Autodesk Fusion 360 part; units mm, degrees
(part 2 of 3)
sketch "Knuckle (2) (2)" plane through (0, 0, 0) normal (1, 0, 0) x (0, 0, -1) in component "Wedgelet_Block_PETG_R"
  line L0 (100, 11) -> (100, 16.5)
  line L1 (100, 16.5) -> (104, 16.5)
  line L2 (104, 16.5) -> (104, 11)
  line L3 (104, 11) -> (100, 11)
extrude "Extrude4'''''" add sketch "Knuckle (2) (2)" along normal blind 4 from surface at 84 bodies 28 in component "Wedgelet_Block_PETG_R"
sketch "Bridge (2)" plane through (0, 0, 0) normal (1, 0, 0) x (0, 0, -1) in component "Wedgelet_Block_PETG_R"
  line L0 (97, 7) -> (97, 10)
  line L1 (97, 10) -> (101, 10)
  line L2 (101, 10) -> (101, 7)
  line L3 (101, 7) -> (97, 7)
extrude "Extrude5'''''" add sketch "Bridge (2)" along normal blind 10 from surface at 70 bodies 28 in component "Wedgelet_Block_PETG_R"
sketch "Rail (2)" plane through (0, 0, 0) normal (1, 0, 0) x (0, 0, -1) in component "Wedgelet_Block_PETG_R"
  line L0 (64, 7) -> (64, 18)
  line L1 (64, 18) -> (98, 18)
  line L2 (98, 18) -> (98, 7)
  line L3 (98, 7) -> (64, 7)
extrude "Extrude6'''''" add sketch "Rail (2)" along normal blind 10 from surface at 70 bodies 28 in component "Wedgelet_Block_PETG_R"
sketch "Pin_Bore (4)" plane through (0, 0, 0) normal (1, 0, 0) x (0, 0, -1) in component "Wedgelet_Block_PETG_R"
  circle A0 centre (102, 14.5) radius 1.6
extrude "Extrude7''''" cut sketch "Pin_Bore (4)" along normal blind 56 from surface at 33 bodies 28 in component "Wedgelet_Block_PETG_R"
sketch "Wall_Insert (2)" plane through (0, 0, 0) normal (1, 0, 0) x (0, 0, -1) in component "Wedgelet_Block_PETG_R"
  circle A0 centre (80, 13.5) radius 2
extrude "Extrude8''''" cut sketch "Wall_Insert (2)" along normal blind 8 from surface at 72 bodies 28 in component "Wedgelet_Block_PETG_R"
sketch "Wall_Insert (1) (2)" plane through (0, 0, 0) normal (1, 0, 0) x (0, 0, -1) in component "Wedgelet_Block_PETG_R"
  circle A0 centre (92, 13.5) radius 2
extrude "Extrude9''''" cut sketch "Wall_Insert (1) (2)" along normal blind 8 from surface at 72 bodies 28 in component "Wedgelet_Block_PETG_R"
sketch "Wedgelet_Carrier_PETG_R1" plane through (0, 0, 0) normal (1, 0, 0) x (0, 0, -1) in component "Wedgelet_Carrier_PETG_R1"
  line L0 (100, 11.5) -> (100, 20.5)
  line L1 (100, 20.5) -> (114, 10.5)
  line L2 (114, 10.5) -> (114, 8)
  line L3 (114, 8) -> (105, 8)
  line L4 (105, 8) -> (104.5, 11.5)
  line L5 (104.5, 11.5) -> (100, 11.5)
extrude "Extrude1''''''''''''''''''''''''''''" add sketch "Wedgelet_Carrier_PETG_R1" along normal blind 20 from surface at 39 separate body makes body 29 in component "Wedgelet_Carrier_PETG_R1"
sketch "Pin_Bore (5)" plane through (0, 0, 0) normal (1, 0, 0) x (0, 0, -1) in component "Wedgelet_Carrier_PETG_R1"
  circle A0 centre (102, 14.5) radius 1.6
extrude "Extrude2'''''''''''''" cut sketch "Pin_Bore (5)" along normal blind 22 from surface at 38 bodies 29 in component "Wedgelet_Carrier_PETG_R1"
sketch "Wedgelet_Insert (3)" plane through (0, 60.8716, -43.4797) normal (0, 0.813733, -0.581238) x (0, 0.581238, 0.813733) in component "Wedgelet_Carrier_PETG_R1"
  line L0 (-86.6626, 39) -> (-69.458, 39)
  line L1 (-69.458, 39) -> (-69.458, 59)
  line L2 (-69.458, 59) -> (-86.6626, 59)
  line L3 (-86.6626, 59) -> (-86.6626, 39)
  circle A0 through (-78.5829, 49, -0.0046) (-81.5829, 50.7321, -0.0046) (-81.5829, 47.2679, -0.0046)
extrude "Extrude3''''''''''" cut sketch "Wedgelet_Insert (3)" along normal mid plane 12 contours A0 in plane through (0, 60.8679, -43.4771) normal (0, 0.813733, -0.581238) bodies 29 in component "Wedgelet_Carrier_PETG_R1"
sketch "Wedgelet_Carrier_PETG_R2" plane through (0, 0, 0) normal (1, 0, 0) x (0, 0, -1) in component "Wedgelet_Carrier_PETG_R2"
  line L0 (100, 11.5) -> (100, 20.5)
  line L1 (100, 20.5) -> (114, 10.5)
  line L2 (114, 10.5) -> (114, 8)
  line L3 (114, 8) -> (105, 8)
  line L4 (105, 8) -> (104.5, 11.5)
  line L5 (104.5, 11.5) -> (100, 11.5)
extrude "Extrude1'''''''''''''''''''''''''''''" add sketch "Wedgelet_Carrier_PETG_R2" along normal blind 16 from surface at 67 separate body makes body 30 in component "Wedgelet_Carrier_PETG_R2"
sketch "Pin_Bore (6)" plane through (0, 0, 0) normal (1, 0, 0) x (0, 0, -1) in component "Wedgelet_Carrier_PETG_R2"
  circle A0 centre (102, 14.5) radius 1.6
extrude "Extrude2''''''''''''''" cut sketch "Pin_Bore (6)" along normal blind 18 from surface at 66 bodies 30 in component "Wedgelet_Carrier_PETG_R2"
sketch "Wedgelet_Insert (4)" plane through (0, 60.8716, -43.4797) normal (0, 0.813733, -0.581238) x (0, 0.581238, 0.813733) in component "Wedgelet_Carrier_PETG_R2"
  line L0 (-86.6626, 67) -> (-69.458, 67)
  line L1 (-69.458, 67) -> (-69.458, 83)
  line L2 (-69.458, 83) -> (-86.6626, 83)
  line L3 (-86.6626, 83) -> (-86.6626, 67)
  circle A0 through (-78.5829, 75, -0.0046) (-81.5829, 76.7321, -0.0046) (-81.5829, 73.2679, -0.0046)
extrude "Extrude3'''''''''''" cut sketch "Wedgelet_Insert (4)" along normal mid plane 12 contours A0 in plane through (0, 60.8679, -43.4771) normal (0, 0.813733, -0.581238) bodies 30 in component "Wedgelet_Carrier_PETG_R2"
sketch "Hinge_Pin_D3_R" plane through (0, 0, 0) normal (1, 0, 0) x (0, 0, -1) in component "Hinge_Pin_D3_R"
  circle A0 centre (102, 14.5) radius 1.5
extrude "Extrude1''''''''''''''''''''''''''''''" add sketch "Hinge_Pin_D3_R" along normal blind 57 from surface at 33.5 separate body makes body 31 in component "Hinge_Pin_D3_R"
sketch "Eclip_Groove (2)" plane through (0, 0, 0) normal (1, 0, 0) x (0, 0, -1) in component "Hinge_Pin_D3_R"
  circle A0 centre (102, 14.5) radius 1.5
  circle A1 centre (102, 14.5) radius 1.15
extrude "Extrude2'''''''''''''''" cut sketch "Eclip_Groove (2)" along normal blind 0.6 from surface at 89 bodies 31 in component "Hinge_Pin_D3_R"
sketch "Eclip_DIN6799_2.3_R" plane through (0, 0, 0) normal (1, 0, 0) x (0, 0, -1) in component "Eclip_DIN6799_2.3_R"
  circle A0 centre (102, 14.5) radius 3.5
  circle A1 centre (102, 14.5) radius 1.15
extrude "Extrude1'''''''''''''''''''''''''''''''" add sketch "Eclip_DIN6799_2.3_R" along normal blind 0.6 from surface at 89 separate body makes body 32 in component "Eclip_DIN6799_2.3_R"
sketch "Sketch1 (8)" plane through (0, 0, 0) normal (0, 1, 0) x (1, 0, 0) in component "Skirt_Plate_1mm_L"
  line L0 (-89.5, -110) -> (-88.5, -110)
  line L1 (-88.5, -110) -> (-88.5, 97)
  line L2 (-88.5, 97) -> (-89.5, 97)
  line L3 (-89.5, 97) -> (-89.5, -110)
extrude "Extrude1''''''''''''''''''''''''''''''''" add sketch "Sketch1 (8)" along normal blind 13 separate body makes body 33 in component "Skirt_Plate_1mm_L"
sketch "Skirt_Wire_D1.5_L" plane through (0, 0, 0) normal (0, 0, 1) x (1, 0, 0) in component "Skirt_Wire_D1.5_L"
  circle A0 centre (-90, 15) radius 0.75
extrude "Extrude1'''''''''''''''''''''''''''''''''" add sketch "Skirt_Wire_D1.5_L" along normal blind 207 from surface at -97 separate body makes body 34 in component "Skirt_Wire_D1.5_L"
sketch "Skirt_Knuckle" plane through (0, 0, 0) normal (1, 0, 0) x (0, 0, -1) in component "Tub_TPU"
  line L0 (-108, 13) -> (-108, 17)
  line L1 (-108, 17) -> (-98, 17)
  line L2 (-98, 17) -> (-98, 13)
  line L3 (-98, 13) -> (-108, 13)
extrude "Extrude42" add sketch "Skirt_Knuckle" along normal blind 4 from surface at -92 bodies 1 in component "Tub_TPU"
sketch "Skirt_Knuckle (1)" plane through (0, 0, 0) normal (1, 0, 0) x (0, 0, -1) in component "Tub_TPU"
  line L0 (-55, 13) -> (-55, 17)
  line L1 (-55, 17) -> (-45, 17)
  line L2 (-45, 17) -> (-45, 13)
  line L3 (-45, 13) -> (-55, 13)
extrude "Extrude43" add sketch "Skirt_Knuckle (1)" along normal blind 4 from surface at -92 bodies 1 in component "Tub_TPU"
sketch "Skirt_Knuckle (2)" plane through (0, 0, 0) normal (1, 0, 0) x (0, 0, -1) in component "Tub_TPU"
  line L0 (0, 13) -> (0, 17)
  line L1 (0, 17) -> (10, 17)
  line L2 (10, 17) -> (10, 13)
  line L3 (10, 13) -> (0, 13)
extrude "Extrude44" add sketch "Skirt_Knuckle (2)" along normal blind 4 from surface at -92 bodies 1 in component "Tub_TPU"
sketch "Skirt_Knuckle (3)" plane through (0, 0, 0) normal (1, 0, 0) x (0, 0, -1) in component "Tub_TPU"
  line L0 (80, 13) -> (80, 17)
  line L1 (80, 17) -> (90, 17)
  line L2 (90, 17) -> (90, 13)
  line L3 (90, 13) -> (80, 13)
extrude "Extrude45" add sketch "Skirt_Knuckle (3)" along normal blind 4 from surface at -92 bodies 1 in component "Tub_TPU"
sketch "Skirt_Wire_Bore" plane through (0, 0, 0) normal (0, 0, 1) x (1, 0, 0) in component "Tub_TPU"
  circle A0 centre (-90, 15) radius 0.8
extrude "Extrude46" cut sketch "Skirt_Wire_Bore" along normal blind 209 from surface at -98 bodies 1 in component "Tub_TPU"
sketch "Sketch1 (9)" plane through (0, 0, 0) normal (0, 1, 0) x (1, 0, 0) in component "Skirt_Clip_PETG_L1"
  line L0 (-92, -90) -> (-89.5, -90)
  line L1 (-89.5, -90) -> (-89.5, -75)
  line L2 (-89.5, -75) -> (-92, -75)
  line L3 (-92, -75) -> (-92, -90)
extrude "Extrude1''''''''''''''''''''''''''''''''''" add sketch "Sketch1 (9)" along normal blind 7 from surface at 10 separate body makes body 35 in component "Skirt_Clip_PETG_L1"
sketch "Wire_Bore" plane through (0, 0, 0) normal (0, 0, 1) x (1, 0, 0) in component "Skirt_Clip_PETG_L1"
  circle A0 centre (-90, 15) radius 0.8
extrude "Extrude2''''''''''''''''" cut sketch "Wire_Bore" along normal blind 17 from surface at 74 bodies 35 in component "Skirt_Clip_PETG_L1"
sketch "M2_Hole" plane through (0, 0, 0) normal (1, 0, 0) x (0, 0, -1) in component "Skirt_Clip_PETG_L1"
  circle A0 centre (-82.5, 11.5) radius 1.1
extrude "Extrude3''''''''''''" cut sketch "M2_Hole" along normal blind 5 from surface at -93 bodies 35 in component "Skirt_Clip_PETG_L1"
sketch "M2_Hole (2)" plane through (0, 0, 0) normal (1, 0, 0) x (0, 0, -1) in component "Skirt_Plate_1mm_L"
  circle A0 centre (-82.5, 11.5) radius 1.1
extrude "Extrude2'''''''''''''''''" cut sketch "M2_Hole (2)" along normal blind 5 from surface at -93 bodies 33 in component "Skirt_Plate_1mm_L"
sketch "Sketch1 (10)" plane through (0, 0, 0) normal (0, 1, 0) x (1, 0, 0) in component "Skirt_Clip_PETG_L2"
  line L0 (-92, -35) -> (-89.5, -35)
  line L1 (-89.5, -35) -> (-89.5, -20)
  line L2 (-89.5, -20) -> (-92, -20)
  line L3 (-92, -20) -> (-92, -35)
extrude "Extrude1'''''''''''''''''''''''''''''''''''" add sketch "Sketch1 (10)" along normal blind 7 from surface at 10 separate body makes body 36 in component "Skirt_Clip_PETG_L2"
sketch "Wire_Bore (2)" plane through (0, 0, 0) normal (0, 0, 1) x (1, 0, 0) in component "Skirt_Clip_PETG_L2"
  circle A0 centre (-90, 15) radius 0.8
extrude "Extrude2''''''''''''''''''" cut sketch "Wire_Bore (2)" along normal blind 17 from surface at 19 bodies 36 in component "Skirt_Clip_PETG_L2"
sketch "M2_Hole (3)" plane through (0, 0, 0) normal (1, 0, 0) x (0, 0, -1) in component "Skirt_Clip_PETG_L2"
  circle A0 centre (-27.5, 11.5) radius 1.1
extrude "Extrude3'''''''''''''" cut sketch "M2_Hole (3)" along normal blind 5 from surface at -93 bodies 36 in component "Skirt_Clip_PETG_L2"
sketch "M2_Hole (1)" plane through (0, 0, 0) normal (1, 0, 0) x (0, 0, -1) in component "Skirt_Plate_1mm_L"
  circle A0 centre (-27.5, 11.5) radius 1.1
extrude "Extrude3''''''''''''''" cut sketch "M2_Hole (1)" along normal blind 5 from surface at -93 bodies 33 in component "Skirt_Plate_1mm_L"
sketch "Sketch1 (11)" plane through (0, 0, 0) normal (0, 1, 0) x (1, 0, 0) in component "Skirt_Clip_PETG_L3"
  line L0 (-92, 25) -> (-89.5, 25)
  line L1 (-89.5, 25) -> (-89.5, 40)
  line L2 (-89.5, 40) -> (-92, 40)
  line L3 (-92, 40) -> (-92, 25)
extrude "Extrude1''''''''''''''''''''''''''''''''''''" add sketch "Sketch1 (11)" along normal blind 7 from surface at 10 separate body makes body 37 in component "Skirt_Clip_PETG_L3"
sketch "Wire_Bore (3)" plane through (0, 0, 0) normal (0, 0, 1) x (1, 0, 0) in component "Skirt_Clip_PETG_L3"
  circle A0 centre (-90, 15) radius 0.8
extrude "Extrude2'''''''''''''''''''" cut sketch "Wire_Bore (3)" along normal blind 17 from surface at -41 bodies 37 in component "Skirt_Clip_PETG_L3"
sketch "M2_Hole (4)" plane through (0, 0, 0) normal (1, 0, 0) x (0, 0, -1) in component "Skirt_Clip_PETG_L3"
  circle A0 centre (32.5, 11.5) radius 1.1
extrude "Extrude3'''''''''''''''" cut sketch "M2_Hole (4)" along normal blind 5 from surface at -93 bodies 37 in component "Skirt_Clip_PETG_L3"
sketch "M2_Hole (2) (2)" plane through (0, 0, 0) normal (1, 0, 0) x (0, 0, -1) in component "Skirt_Plate_1mm_L"
  circle A0 centre (32.5, 11.5) radius 1.1
extrude "Extrude4''''''" cut sketch "M2_Hole (2) (2)" along normal blind 5 from surface at -93 bodies 33 in component "Skirt_Plate_1mm_L"
sketch "Sketch1 (12)" plane through (0, 0, 0) normal (0, 1, 0) x (1, 0, 0) in component "Skirt_Clip_PETG_L4"
  line L0 (-92, 55) -> (-89.5, 55)
  line L1 (-89.5, 55) -> (-89.5, 70)
  line L2 (-89.5, 70) -> (-92, 70)
  line L3 (-92, 70) -> (-92, 55)
extrude "Extrude1'''''''''''''''''''''''''''''''''''''" add sketch "Sketch1 (12)" along normal blind 7 from surface at 10 separate body makes body 38 in component "Skirt_Clip_PETG_L4"
sketch "Wire_Bore (4)" plane through (0, 0, 0) normal (0, 0, 1) x (1, 0, 0) in component "Skirt_Clip_PETG_L4"
  circle A0 centre (-90, 15) radius 0.8
extrude "Extrude2''''''''''''''''''''" cut sketch "Wire_Bore (4)" along normal blind 17 from surface at -71 bodies 38 in component "Skirt_Clip_PETG_L4"
sketch "M2_Hole (5)" plane through (0, 0, 0) normal (1, 0, 0) x (0, 0, -1) in component "Skirt_Clip_PETG_L4"
  circle A0 centre (62.5, 11.5) radius 1.1
extrude "Extrude3''''''''''''''''" cut sketch "M2_Hole (5)" along normal blind 5 from surface at -93 bodies 38 in component "Skirt_Clip_PETG_L4"
sketch "M2_Hole (3) (2)" plane through (0, 0, 0) normal (1, 0, 0) x (0, 0, -1) in component "Skirt_Plate_1mm_L"
  circle A0 centre (62.5, 11.5) radius 1.1
extrude "Extrude5''''''" cut sketch "M2_Hole (3) (2)" along normal blind 5 from surface at -93 bodies 33 in component "Skirt_Plate_1mm_L"
sketch "Sketch1 (13)" plane through (0, 0, 0) normal (0, 1, 0) x (1, 0, 0) in component "Skirt_Plate_1mm_R"
  line L0 (88.5, -110) -> (89.5, -110)
  line L1 (89.5, -110) -> (89.5, 97)
  line L2 (89.5, 97) -> (88.5, 97)
  line L3 (88.5, 97) -> (88.5, -110)
extrude "Extrude1''''''''''''''''''''''''''''''''''''''" add sketch "Sketch1 (13)" along normal blind 13 separate body makes body 39 in component "Skirt_Plate_1mm_R"
sketch "Skirt_Wire_D1.5_R" plane through (0, 0, 0) normal (0, 0, 1) x (1, 0, 0) in component "Skirt_Wire_D1.5_R"
  circle A0 centre (90, 15) radius 0.75
extrude "Extrude1'''''''''''''''''''''''''''''''''''''''" add sketch "Skirt_Wire_D1.5_R" along normal blind 207 from surface at -97 separate body makes body 40 in component "Skirt_Wire_D1.5_R"
sketch "Skirt_Knuckle (4)" plane through (0, 0, 0) normal (1, 0, 0) x (0, 0, -1) in component "Tub_TPU"
  line L0 (-108, 13) -> (-108, 17)
  line L1 (-108, 17) -> (-98, 17)
  line L2 (-98, 17) -> (-98, 13)
  line L3 (-98, 13) -> (-108, 13)
extrude "Extrude47" add sketch "Skirt_Knuckle (4)" along normal blind 4 from surface at 88 bodies 1 in component "Tub_TPU"
sketch "Skirt_Knuckle (5)" plane through (0, 0, 0) normal (1, 0, 0) x (0, 0, -1) in component "Tub_TPU"
  line L0 (-55, 13) -> (-55, 17)
  line L1 (-55, 17) -> (-45, 17)
  line L2 (-45, 17) -> (-45, 13)
  line L3 (-45, 13) -> (-55, 13)
extrude "Extrude48" add sketch "Skirt_Knuckle (5)" along normal blind 4 from surface at 88 bodies 1 in component "Tub_TPU"
sketch "Skirt_Knuckle (6)" plane through (0, 0, 0) normal (1, 0, 0) x (0, 0, -1) in component "Tub_TPU"
  line L0 (0, 13) -> (0, 17)
  line L1 (0, 17) -> (10, 17)
  line L2 (10, 17) -> (10, 13)
  line L3 (10, 13) -> (0, 13)
extrude "Extrude49" add sketch "Skirt_Knuckle (6)" along normal blind 4 from surface at 88 bodies 1 in component "Tub_TPU"
sketch "Skirt_Knuckle (7)" plane through (0, 0, 0) normal (1, 0, 0) x (0, 0, -1) in component "Tub_TPU"
  line L0 (80, 13) -> (80, 17)
  line L1 (80, 17) -> (90, 17)
  line L2 (90, 17) -> (90, 13)
  line L3 (90, 13) -> (80, 13)
extrude "Extrude50" add sketch "Skirt_Knuckle (7)" along normal blind 4 from surface at 88 bodies 1 in component "Tub_TPU"
sketch "Skirt_Wire_Bore (1)" plane through (0, 0, 0) normal (0, 0, 1) x (1, 0, 0) in component "Tub_TPU"
  circle A0 centre (90, 15) radius 0.8
extrude "Extrude51" cut sketch "Skirt_Wire_Bore (1)" along normal blind 209 from surface at -98 bodies 1 in component "Tub_TPU"
sketch "Sketch1 (14)" plane through (0, 0, 0) normal (0, 1, 0) x (1, 0, 0) in component "Skirt_Clip_PETG_R1"
  line L0 (89.5, -90) -> (92, -90)
  line L1 (92, -90) -> (92, -75)
  line L2 (92, -75) -> (89.5, -75)
  line L3 (89.5, -75) -> (89.5, -90)
extrude "Extrude1''''''''''''''''''''''''''''''''''''''''" add sketch "Sketch1 (14)" along normal blind 7 from surface at 10 separate body makes body 41 in component "Skirt_Clip_PETG_R1"
sketch "Wire_Bore (5)" plane through (0, 0, 0) normal (0, 0, 1) x (1, 0, 0) in component "Skirt_Clip_PETG_R1"
  circle A0 centre (90, 15) radius 0.8
extrude "Extrude2'''''''''''''''''''''" cut sketch "Wire_Bore (5)" along normal blind 17 from surface at 74 bodies 41 in component "Skirt_Clip_PETG_R1"
sketch "M2_Hole (6)" plane through (0, 0, 0) normal (1, 0, 0) x (0, 0, -1) in component "Skirt_Clip_PETG_R1"
  circle A0 centre (-82.5, 11.5) radius 1.1
extrude "Extrude3'''''''''''''''''" cut sketch "M2_Hole (6)" along normal blind 5 from surface at 88 bodies 41 in component "Skirt_Clip_PETG_R1"
sketch "M2_Hole (7)" plane through (0, 0, 0) normal (1, 0, 0) x (0, 0, -1) in component "Skirt_Plate_1mm_R"
  circle A0 centre (-82.5, 11.5) radius 1.1
extrude "Extrude2''''''''''''''''''''''" cut sketch "M2_Hole (7)" along normal blind 5 from surface at 88 bodies 39 in component "Skirt_Plate_1mm_R"
sketch "Sketch1 (15)" plane through (0, 0, 0) normal (0, 1, 0) x (1, 0, 0) in component "Skirt_Clip_PETG_R2"
  line L0 (89.5, -35) -> (92, -35)
  line L1 (92, -35) -> (92, -20)
  line L2 (92, -20) -> (89.5, -20)
  line L3 (89.5, -20) -> (89.5, -35)
extrude "Extrude1'''''''''''''''''''''''''''''''''''''''''" add sketch "Sketch1 (15)" along normal blind 7 from surface at 10 separate body makes body 42 in component "Skirt_Clip_PETG_R2"
sketch "Wire_Bore (6)" plane through (0, 0, 0) normal (0, 0, 1) x (1, 0, 0) in component "Skirt_Clip_PETG_R2"
  circle A0 centre (90, 15) radius 0.8
extrude "Extrude2'''''''''''''''''''''''" cut sketch "Wire_Bore (6)" along normal blind 17 from surface at 19 bodies 42 in component "Skirt_Clip_PETG_R2"
sketch "M2_Hole (8)" plane through (0, 0, 0) normal (1, 0, 0) x (0, 0, -1) in component "Skirt_Clip_PETG_R2"
  circle A0 centre (-27.5, 11.5) radius 1.1
extrude "Extrude3''''''''''''''''''" cut sketch "M2_Hole (8)" along normal blind 5 from surface at 88 bodies 42 in component "Skirt_Clip_PETG_R2"
sketch "M2_Hole (1) (2)" plane through (0, 0, 0) normal (1, 0, 0) x (0, 0, -1) in component "Skirt_Plate_1mm_R"
  circle A0 centre (-27.5, 11.5) radius 1.1
extrude "Extrude3'''''''''''''''''''" cut sketch "M2_Hole (1) (2)" along normal blind 5 from surface at 88 bodies 39 in component "Skirt_Plate_1mm_R"
sketch "Sketch1 (16)" plane through (0, 0, 0) normal (0, 1, 0) x (1, 0, 0) in component "Skirt_Clip_PETG_R3"
  line L0 (89.5, 25) -> (92, 25)
  line L1 (92, 25) -> (92, 40)
  line L2 (92, 40) -> (89.5, 40)
  line L3 (89.5, 40) -> (89.5, 25)
extrude "Extrude1''''''''''''''''''''''''''''''''''''''''''" add sketch "Sketch1 (16)" along normal blind 7 from surface at 10 separate body makes body 43 in component "Skirt_Clip_PETG_R3"
sketch "Wire_Bore (7)" plane through (0, 0, 0) normal (0, 0, 1) x (1, 0, 0) in component "Skirt_Clip_PETG_R3"
  circle A0 centre (90, 15) radius 0.8
extrude "Extrude2''''''''''''''''''''''''" cut sketch "Wire_Bore (7)" along normal blind 17 from surface at -41 bodies 43 in component "Skirt_Clip_PETG_R3"
sketch "M2_Hole (9)" plane through (0, 0, 0) normal (1, 0, 0) x (0, 0, -1) in component "Skirt_Clip_PETG_R3"
  circle A0 centre (32.5, 11.5) radius 1.1
extrude "Extrude3''''''''''''''''''''" cut sketch "M2_Hole (9)" along normal blind 5 from surface at 88 bodies 43 in component "Skirt_Clip_PETG_R3"
sketch "M2_Hole (2) (3)" plane through (0, 0, 0) normal (1, 0, 0) x (0, 0, -1) in component "Skirt_Plate_1mm_R"
  circle A0 centre (32.5, 11.5) radius 1.1
extrude "Extrude4'''''''" cut sketch "M2_Hole (2) (3)" along normal blind 5 from surface at 88 bodies 39 in component "Skirt_Plate_1mm_R"
sketch "Sketch1 (17)" plane through (0, 0, 0) normal (0, 1, 0) x (1, 0, 0) in component "Skirt_Clip_PETG_R4"
  line L0 (89.5, 55) -> (92, 55)
  line L1 (92, 55) -> (92, 70)
  line L2 (92, 70) -> (89.5, 70)
  line L3 (89.5, 70) -> (89.5, 55)
extrude "Extrude1'''''''''''''''''''''''''''''''''''''''''''" add sketch "Sketch1 (17)" along normal blind 7 from surface at 10 separate body makes body 44 in component "Skirt_Clip_PETG_R4"
sketch "Wire_Bore (8)" plane through (0, 0, 0) normal (0, 0, 1) x (1, 0, 0) in component "Skirt_Clip_PETG_R4"
  circle A0 centre (90, 15) radius 0.8
extrude "Extrude2'''''''''''''''''''''''''" cut sketch "Wire_Bore (8)" along normal blind 17 from surface at -71 bodies 44 in component "Skirt_Clip_PETG_R4"
sketch "M2_Hole (10)" plane through (0, 0, 0) normal (1, 0, 0) x (0, 0, -1) in component "Skirt_Clip_PETG_R4"
  circle A0 centre (62.5, 11.5) radius 1.1
extrude "Extrude3'''''''''''''''''''''" cut sketch "M2_Hole (10)" along normal blind 5 from surface at 88 bodies 44 in component "Skirt_Clip_PETG_R4"
sketch "M2_Hole (3) (3)" plane through (0, 0, 0) normal (1, 0, 0) x (0, 0, -1) in component "Skirt_Plate_1mm_R"
  circle A0 centre (62.5, 11.5) radius 1.1
extrude "Extrude5'''''''" cut sketch "M2_Hole (3) (3)" along normal blind 5 from surface at 88 bodies 39 in component "Skirt_Plate_1mm_R"
sketch "Sketch1 (18)" plane through (0, 0, 0) normal (0, 1, 0) x (1, 0, 0) in component "Skirt_Plate_1mm_Rear"
  line L0 (-88, -111.5) -> (88, -111.5)
  line L1 (88, -111.5) -> (88, -110.5)
  line L2 (88, -110.5) -> (-88, -110.5)
  line L3 (-88, -110.5) -> (-88, -111.5)
extrude "Extrude1''''''''''''''''''''''''''''''''''''''''''''" add sketch "Sketch1 (18)" along normal blind 13 separate body makes body 45 in component "Skirt_Plate_1mm_Rear"
sketch "Skirt_Wire_D1.5_Rear" plane through (0, 0, 0) normal (1, 0, 0) x (0, 0, -1) in component "Skirt_Wire_D1.5_Rear"
  circle A0 centre (-112, 15) radius 0.75
extrude "Extrude1'''''''''''''''''''''''''''''''''''''''''''''" add sketch "Skirt_Wire_D1.5_Rear" along normal blind 176 from surface at -88 separate body makes body 46 in component "Skirt_Wire_D1.5_Rear"
sketch "Skirt_Knuckle (8)" plane through (0, 0, 0) normal (1, 0, 0) x (0, 0, -1) in component "Tub_TPU"
  line L0 (-114, 13) -> (-114, 17)
  line L1 (-114, 17) -> (-110, 17)
  line L2 (-110, 17) -> (-110, 13)
  line L3 (-110, 13) -> (-114, 13)
extrude "Extrude52" add sketch "Skirt_Knuckle (8)" along normal blind 10 from surface at -86 bodies 1 in component "Tub_TPU"
sketch "Skirt_Knuckle (9)" plane through (0, 0, 0) normal (1, 0, 0) x (0, 0, -1) in component "Tub_TPU"
  line L0 (-114, 13) -> (-114, 17)
  line L1 (-114, 17) -> (-110, 17)
  line L2 (-110, 17) -> (-110, 13)
  line L3 (-110, 13) -> (-114, 13)
extrude "Extrude53" add sketch "Skirt_Knuckle (9)" along normal blind 10 from surface at -30 bodies 1 in component "Tub_TPU"
sketch "Skirt_Knuckle (10)" plane through (0, 0, 0) normal (1, 0, 0) x (0, 0, -1) in component "Tub_TPU"
  line L0 (-114, 13) -> (-114, 17)
  line L1 (-114, 17) -> (-110, 17)
  line L2 (-110, 17) -> (-110, 13)
  line L3 (-110, 13) -> (-114, 13)
extrude "Extrude54" add sketch "Skirt_Knuckle (10)" along normal blind 10 from surface at 20 bodies 1 in component "Tub_TPU"
sketch "Skirt_Knuckle (11)" plane through (0, 0, 0) normal (1, 0, 0) x (0, 0, -1) in component "Tub_TPU"
  line L0 (-114, 13) -> (-114, 17)
  line L1 (-114, 17) -> (-110, 17)
  line L2 (-110, 17) -> (-110, 13)
  line L3 (-110, 13) -> (-114, 13)
extrude "Extrude55" add sketch "Skirt_Knuckle (11)" along normal blind 10 from surface at 76 bodies 1 in component "Tub_TPU"
sketch "Skirt_Wire_Bore (2)" plane through (0, 0, 0) normal (1, 0, 0) x (0, 0, -1) in component "Tub_TPU"
  circle A0 centre (-112, 15) radius 0.8
extrude "Extrude56" cut sketch "Skirt_Wire_Bore (2)" along normal blind 178 from surface at -89 bodies 1 in component "Tub_TPU"
sketch "Sketch1 (19)" plane through (0, 0, 0) normal (0, 1, 0) x (1, 0, 0) in component "Skirt_Clip_PETG_Rear1"
  line L0 (-65, -114) -> (-50, -114)
  line L1 (-50, -114) -> (-50, -111.5)
  line L2 (-50, -111.5) -> (-65, -111.5)
  line L3 (-65, -111.5) -> (-65, -114)
extrude "Extrude1''''''''''''''''''''''''''''''''''''''''''''''" add sketch "Sketch1 (19)" along normal blind 7 from surface at 10 separate body makes body 47 in component "Skirt_Clip_PETG_Rear1"
sketch "Wire_Bore (9)" plane through (0, 0, 0) normal (1, 0, 0) x (0, 0, -1) in component "Skirt_Clip_PETG_Rear1"
  circle A0 centre (-112, 15) radius 0.8
extrude "Extrude2''''''''''''''''''''''''''" cut sketch "Wire_Bore (9)" along normal blind 17 from surface at -66 bodies 47 in component "Skirt_Clip_PETG_Rear1"
sketch "M2_Hole (11)" plane through (0, 0, 0) normal (0, 0, 1) x (1, 0, 0) in component "Skirt_Clip_PETG_Rear1"
  circle A0 centre (-57.5, 11.5) radius 1.1
extrude "Extrude3''''''''''''''''''''''" cut sketch "M2_Hole (11)" along normal blind 5 from surface at 110 bodies 47 in component "Skirt_Clip_PETG_Rear1"
sketch "M2_Hole (12)" plane through (0, 0, 0) normal (0, 0, 1) x (1, 0, 0) in component "Skirt_Plate_1mm_Rear"
  circle A0 centre (-57.5, 11.5) radius 1.1
extrude "Extrude2'''''''''''''''''''''''''''" cut sketch "M2_Hole (12)" along normal blind 5 from surface at 110 bodies 45 in component "Skirt_Plate_1mm_Rear"
sketch "Sketch1 (20)" plane through (0, 0, 0) normal (0, 1, 0) x (1, 0, 0) in component "Skirt_Clip_PETG_Rear2"
  line L0 (-8, -114) -> (8, -114)
  line L1 (8, -114) -> (8, -111.5)
  line L2 (8, -111.5) -> (-8, -111.5)
  line L3 (-8, -111.5) -> (-8, -114)
extrude "Extrude1'''''''''''''''''''''''''''''''''''''''''''''''" add sketch "Sketch1 (20)" along normal blind 7 from surface at 10 separate body makes body 48 in component "Skirt_Clip_PETG_Rear2"
sketch "Wire_Bore (10)" plane through (0, 0, 0) normal (1, 0, 0) x (0, 0, -1) in component "Skirt_Clip_PETG_Rear2"
  circle A0 centre (-112, 15) radius 0.8
extrude "Extrude2''''''''''''''''''''''''''''" cut sketch "Wire_Bore (10)" along normal blind 18 from surface at -9 bodies 48 in component "Skirt_Clip_PETG_Rear2"
sketch "M2_Hole (13)" plane through (0, 0, 0) normal (0, 0, 1) x (1, 0, 0) in component "Skirt_Clip_PETG_Rear2"
  circle A0 centre (0, 11.5) radius 1.1
extrude "Extrude3'''''''''''''''''''''''" cut sketch "M2_Hole (13)" along normal blind 5 from surface at 110 bodies 48 in component "Skirt_Clip_PETG_Rear2"
sketch "M2_Hole (1) (3)" plane through (0, 0, 0) normal (0, 0, 1) x (1, 0, 0) in component "Skirt_Plate_1mm_Rear"
  circle A0 centre (0, 11.5) radius 1.1
extrude "Extrude3''''''''''''''''''''''''" cut sketch "M2_Hole (1) (3)" along normal blind 5 from surface at 110 bodies 45 in component "Skirt_Plate_1mm_Rear"
sketch "Sketch1 (21)" plane through (0, 0, 0) normal (0, 1, 0) x (1, 0, 0) in component "Skirt_Clip_PETG_Rear3"
  line L0 (50, -114) -> (65, -114)
  line L1 (65, -114) -> (65, -111.5)
  line L2 (65, -111.5) -> (50, -111.5)
  line L3 (50, -111.5) -> (50, -114)
extrude "Extrude1''''''''''''''''''''''''''''''''''''''''''''''''" add sketch "Sketch1 (21)" along normal blind 7 from surface at 10 separate body makes body 49 in component "Skirt_Clip_PETG_Rear3"
sketch "Wire_Bore (11)" plane through (0, 0, 0) normal (1, 0, 0) x (0, 0, -1) in component "Skirt_Clip_PETG_Rear3"
  circle A0 centre (-112, 15) radius 0.8
extrude "Extrude2'''''''''''''''''''''''''''''" cut sketch "Wire_Bore (11)" along normal blind 17 from surface at 49 bodies 49 in component "Skirt_Clip_PETG_Rear3"
sketch "M2_Hole (14)" plane through (0, 0, 0) normal (0, 0, 1) x (1, 0, 0) in component "Skirt_Clip_PETG_Rear3"
  circle A0 centre (57.5, 11.5) radius 1.1
extrude "Extrude3'''''''''''''''''''''''''" cut sketch "M2_Hole (14)" along normal blind 5 from surface at 110 bodies 49 in component "Skirt_Clip_PETG_Rear3"
sketch "M2_Hole (2) (4)" plane through (0, 0, 0) normal (0, 0, 1) x (1, 0, 0) in component "Skirt_Plate_1mm_Rear"
  circle A0 centre (57.5, 11.5) radius 1.1
extrude "Extrude4''''''''" cut sketch "M2_Hole (2) (4)" along normal blind 5 from surface at 110 bodies 45 in component "Skirt_Plate_1mm_Rear"
sketch "JGA25_370_400rpm_Front_L" plane through (0, 0, 0) normal (1, 0, 0) x (0, 0, -1) in component "JGA25_370_400rpm_Front_L"
  circle A0 centre (10, 32) radius 12.5
extrude "Extrude1'''''''''''''''''''''''''''''''''''''''''''''''''" add sketch "JGA25_370_400rpm_Front_L" along normal blind 52 from surface at -56 separate body makes body 50 in component "JGA25_370_400rpm_Front_L"
sketch "Wheel_Hub_PETG_Front_L" plane through (0, 0, 0) normal (1, 0, 0) x (0, 0, -1) in component "Wheel_Hub_PETG_Front_L"
  circle A0 centre (10, 32) radius 22
  line L0 (11.55, 32) -> (11.55, 32.356)
  line L1 (11.55, 32.356) -> (11.55, 32.7011)
  line L2 (11.55, 32.7011) -> (11.55, 33.025)
  line L3 (11.55, 33.025) -> (11.55, 33.3177)
  line L4 (11.55, 33.3177) -> (11.3177, 33.5704)
  line L5 (11.3177, 33.5704) -> (11.025, 33.7754)
  line L6 (11.025, 33.7754) -> (10.7011, 33.9264)
  line L7 (10.7011, 33.9264) -> (10.356, 34.0189)
  line L8 (10.356, 34.0189) -> (10, 34.05)
  line L9 (10, 34.05) -> (9.644, 34.0189)
  line L10 (9.644, 34.0189) -> (9.2989, 33.9264)
  line L11 (9.2989, 33.9264) -> (8.975, 33.7754)
  line L12 (8.975, 33.7754) -> (8.6823, 33.5704)
  line L13 (8.6823, 33.5704) -> (8.4296, 33.3177)
  line L14 (8.4296, 33.3177) -> (8.2246, 33.025)
  line L15 (8.2246, 33.025) -> (8.0736, 32.7011)
  line L16 (8.0736, 32.7011) -> (7.9811, 32.356)
  line L17 (7.9811, 32.356) -> (7.95, 32)
  line L18 (7.95, 32) -> (7.9811, 31.644)
  line L19 (7.9811, 31.644) -> (8.0736, 31.2989)
  line L20 (8.0736, 31.2989) -> (8.2246, 30.975)
  line L21 (8.2246, 30.975) -> (8.4296, 30.6823)
  line L22 (8.4296, 30.6823) -> (8.6823, 30.4296)
  line L23 (8.6823, 30.4296) -> (8.975, 30.2246)
  line L24 (8.975, 30.2246) -> (9.2989, 30.0736)
  line L25 (9.2989, 30.0736) -> (9.644, 29.9811)
  line L26 (9.644, 29.9811) -> (10, 29.95)
  line L27 (10, 29.95) -> (10.356, 29.9811)
  line L28 (10.356, 29.9811) -> (10.7011, 30.0736)
  line L29 (10.7011, 30.0736) -> (11.025, 30.2246)
  line L30 (11.025, 30.2246) -> (11.3177, 30.4296)
  line L31 (11.3177, 30.4296) -> (11.55, 30.6823)
  line L32 (11.55, 30.6823) -> (11.55, 30.975)
  line L33 (11.55, 30.975) -> (11.55, 31.2989)
  line L34 (11.55, 31.2989) -> (11.55, 31.644)
  line L35 (11.55, 31.644) -> (11.55, 32)
  circle A1 centre (23, 32) radius 4
  circle A2 centre (14.0172, 44.3637) radius 4
  circle A3 centre (-0.5172, 39.6412) radius 4
  circle A4 centre (-0.5172, 24.3588) radius 4
  circle A5 centre (14.0172, 19.6363) radius 4
extrude "Extrude1''''''''''''''''''''''''''''''''''''''''''''''''''" add sketch "Wheel_Hub_PETG_Front_L" along normal blind 16 from surface at -78 separate body makes body 51 in component "Wheel_Hub_PETG_Front_L"
sketch "Wheel_Tyre_TPU_Front_L" plane through (0, 0, 0) normal (1, 0, 0) x (0, 0, -1) in component "Wheel_Tyre_TPU_Front_L"
  circle A0 centre (10, 32) radius 32
  circle A1 centre (10, 32) radius 22
extrude "Extrude1'''''''''''''''''''''''''''''''''''''''''''''''''''" add sketch "Wheel_Tyre_TPU_Front_L" along normal blind 16 from surface at -78 separate body makes body 52 in component "Wheel_Tyre_TPU_Front_L"
sketch "JGA25_370_400rpm_Front_R" plane through (0, 0, 0) normal (1, 0, 0) x (0, 0, -1) in component "JGA25_370_400rpm_Front_R"
  circle A0 centre (10, 32) radius 12.5
extrude "Extrude1''''''''''''''''''''''''''''''''''''''''''''''''''''" add sketch "JGA25_370_400rpm_Front_R" along normal blind 52 from surface at 4 separate body makes body 53 in component "JGA25_370_400rpm_Front_R"
sketch "Wheel_Hub_PETG_Front_R" plane through (0, 0, 0) normal (1, 0, 0) x (0, 0, -1) in component "Wheel_Hub_PETG_Front_R"
  circle A0 centre (10, 32) radius 22
  line L0 (11.55, 32) -> (11.55, 32.356)
  line L1 (11.55, 32.356) -> (11.55, 32.7011)
  line L2 (11.55, 32.7011) -> (11.55, 33.025)
  line L3 (11.55, 33.025) -> (11.55, 33.3177)
  line L4 (11.55, 33.3177) -> (11.3177, 33.5704)
  line L5 (11.3177, 33.5704) -> (11.025, 33.7754)
  line L6 (11.025, 33.7754) -> (10.7011, 33.9264)
  line L7 (10.7011, 33.9264) -> (10.356, 34.0189)
  line L8 (10.356, 34.0189) -> (10, 34.05)
  line L9 (10, 34.05) -> (9.644, 34.0189)
  line L10 (9.644, 34.0189) -> (9.2989, 33.9264)
  line L11 (9.2989, 33.9264) -> (8.975, 33.7754)
  line L12 (8.975, 33.7754) -> (8.6823, 33.5704)
  line L13 (8.6823, 33.5704) -> (8.4296, 33.3177)
  line L14 (8.4296, 33.3177) -> (8.2246, 33.025)
  line L15 (8.2246, 33.025) -> (8.0736, 32.7011)
  line L16 (8.0736, 32.7011) -> (7.9811, 32.356)
  line L17 (7.9811, 32.356) -> (7.95, 32)
  line L18 (7.95, 32) -> (7.9811, 31.644)
  line L19 (7.9811, 31.644) -> (8.0736, 31.2989)
  line L20 (8.0736, 31.2989) -> (8.2246, 30.975)
  line L21 (8.2246, 30.975) -> (8.4296, 30.6823)
  line L22 (8.4296, 30.6823) -> (8.6823, 30.4296)
  line L23 (8.6823, 30.4296) -> (8.975, 30.2246)
  line L24 (8.975, 30.2246) -> (9.2989, 30.0736)
  line L25 (9.2989, 30.0736) -> (9.644, 29.9811)
  line L26 (9.644, 29.9811) -> (10, 29.95)
  line L27 (10, 29.95) -> (10.356, 29.9811)
  line L28 (10.356, 29.9811) -> (10.7011, 30.0736)
  line L29 (10.7011, 30.0736) -> (11.025, 30.2246)
  line L30 (11.025, 30.2246) -> (11.3177, 30.4296)
  line L31 (11.3177, 30.4296) -> (11.55, 30.6823)
  line L32 (11.55, 30.6823) -> (11.55, 30.975)
  line L33 (11.55, 30.975) -> (11.55, 31.2989)
  line L34 (11.55, 31.2989) -> (11.55, 31.644)
  line L35 (11.55, 31.644) -> (11.55, 32)
  circle A1 centre (23, 32) radius 4
  circle A2 centre (14.0172, 44.3637) radius 4
  circle A3 centre (-0.5172, 39.6412) radius 4
  circle A4 centre (-0.5172, 24.3588) radius 4
  circle A5 centre (14.0172, 19.6363) radius 4
extrude "Extrude1'''''''''''''''''''''''''''''''''''''''''''''''''''''" add sketch "Wheel_Hub_PETG_Front_R" along normal blind 16 from surface at 62 separate body makes body 54 in component "Wheel_Hub_PETG_Front_R"
sketch "Wheel_Tyre_TPU_Front_R" plane through (0, 0, 0) normal (1, 0, 0) x (0, 0, -1) in component "Wheel_Tyre_TPU_Front_R"
  circle A0 centre (10, 32) radius 32
  circle A1 centre (10, 32) radius 22
extrude "Extrude1''''''''''''''''''''''''''''''''''''''''''''''''''''''" add sketch "Wheel_Tyre_TPU_Front_R" along normal blind 16 from surface at 62 separate body makes body 55 in component "Wheel_Tyre_TPU_Front_R"
sketch "JGA25_370_400rpm_Rear_L" plane through (0, 0, 0) normal (1, 0, 0) x (0, 0, -1) in component "JGA25_370_400rpm_Rear_L"
  circle A0 centre (-70, 32) radius 12.5
extrude "Extrude1'''''''''''''''''''''''''''''''''''''''''''''''''''''''" add sketch "JGA25_370_400rpm_Rear_L" along normal blind 52 from surface at -56 separate body makes body 56 in component "JGA25_370_400rpm_Rear_L"
sketch "Wheel_Hub_PETG_Rear_L" plane through (0, 0, 0) normal (1, 0, 0) x (0, 0, -1) in component "Wheel_Hub_PETG_Rear_L"
  circle A0 centre (-70, 32) radius 22
  line L0 (-68.45, 32) -> (-68.45, 32.356)
  line L1 (-68.45, 32.356) -> (-68.45, 32.7011)
  line L2 (-68.45, 32.7011) -> (-68.45, 33.025)
  line L3 (-68.45, 33.025) -> (-68.45, 33.3177)
  line L4 (-68.45, 33.3177) -> (-68.6823, 33.5704)
  line L5 (-68.6823, 33.5704) -> (-68.975, 33.7754)
  line L6 (-68.975, 33.7754) -> (-69.2989, 33.9264)
  line L7 (-69.2989, 33.9264) -> (-69.644, 34.0189)
  line L8 (-69.644, 34.0189) -> (-70, 34.05)
  line L9 (-70, 34.05) -> (-70.356, 34.0189)
  line L10 (-70.356, 34.0189) -> (-70.7011, 33.9264)
  line L11 (-70.7011, 33.9264) -> (-71.025, 33.7754)
  line L12 (-71.025, 33.7754) -> (-71.3177, 33.5704)
  line L13 (-71.3177, 33.5704) -> (-71.5704, 33.3177)
  line L14 (-71.5704, 33.3177) -> (-71.7754, 33.025)
  line L15 (-71.7754, 33.025) -> (-71.9264, 32.7011)
  line L16 (-71.9264, 32.7011) -> (-72.0189, 32.356)
  line L17 (-72.0189, 32.356) -> (-72.05, 32)
  line L18 (-72.05, 32) -> (-72.0189, 31.644)
  line L19 (-72.0189, 31.644) -> (-71.9264, 31.2989)
  line L20 (-71.9264, 31.2989) -> (-71.7754, 30.975)
  line L21 (-71.7754, 30.975) -> (-71.5704, 30.6823)
  line L22 (-71.5704, 30.6823) -> (-71.3177, 30.4296)
  line L23 (-71.3177, 30.4296) -> (-71.025, 30.2246)
  line L24 (-71.025, 30.2246) -> (-70.7011, 30.0736)
  line L25 (-70.7011, 30.0736) -> (-70.356, 29.9811)
  line L26 (-70.356, 29.9811) -> (-70, 29.95)
  line L27 (-70, 29.95) -> (-69.644, 29.9811)
  line L28 (-69.644, 29.9811) -> (-69.2989, 30.0736)
  line L29 (-69.2989, 30.0736) -> (-68.975, 30.2246)
  line L30 (-68.975, 30.2246) -> (-68.6823, 30.4296)
  line L31 (-68.6823, 30.4296) -> (-68.45, 30.6823)
  line L32 (-68.45, 30.6823) -> (-68.45, 30.975)
  line L33 (-68.45, 30.975) -> (-68.45, 31.2989)
  line L34 (-68.45, 31.2989) -> (-68.45, 31.644)
  line L35 (-68.45, 31.644) -> (-68.45, 32)
  circle A1 centre (-57, 32) radius 4
  circle A2 centre (-65.9828, 44.3637) radius 4
  circle A3 centre (-80.5172, 39.6412) radius 4
  circle A4 centre (-80.5172, 24.3588) radius 4
  circle A5 centre (-65.9828, 19.6363) radius 4
extrude "Extrude1''''''''''''''''''''''''''''''''''''''''''''''''''''''''" add sketch "Wheel_Hub_PETG_Rear_L" along normal blind 16 from surface at -78 separate body makes body 57 in component "Wheel_Hub_PETG_Rear_L"
sketch "Wheel_Tyre_TPU_Rear_L" plane through (0, 0, 0) normal (1, 0, 0) x (0, 0, -1) in component "Wheel_Tyre_TPU_Rear_L"
  circle A0 centre (-70, 32) radius 32
  circle A1 centre (-70, 32) radius 22
extrude "Extrude1'''''''''''''''''''''''''''''''''''''''''''''''''''''''''" add sketch "Wheel_Tyre_TPU_Rear_L" along normal blind 16 from surface at -78 separate body makes body 58 in component "Wheel_Tyre_TPU_Rear_L"
sketch "JGA25_370_400rpm_Rear_R" plane through (0, 0, 0) normal (1, 0, 0) x (0, 0, -1) in component "JGA25_370_400rpm_Rear_R"
  circle A0 centre (-70, 32) radius 12.5
extrude "Extrude1''''''''''''''''''''''''''''''''''''''''''''''''''''''''''" add sketch "JGA25_370_400rpm_Rear_R" along normal blind 52 from surface at 4 separate body makes body 59 in component "JGA25_370_400rpm_Rear_R"
sketch "Wheel_Hub_PETG_Rear_R" plane through (0, 0, 0) normal (1, 0, 0) x (0, 0, -1) in component "Wheel_Hub_PETG_Rear_R"
  circle A0 centre (-70, 32) radius 22
  line L0 (-68.45, 32) -> (-68.45, 32.356)
  line L1 (-68.45, 32.356) -> (-68.45, 32.7011)
  line L2 (-68.45, 32.7011) -> (-68.45, 33.025)
  line L3 (-68.45, 33.025) -> (-68.45, 33.3177)
  line L4 (-68.45, 33.3177) -> (-68.6823, 33.5704)
  line L5 (-68.6823, 33.5704) -> (-68.975, 33.7754)
  line L6 (-68.975, 33.7754) -> (-69.2989, 33.9264)
  line L7 (-69.2989, 33.9264) -> (-69.644, 34.0189)
  line L8 (-69.644, 34.0189) -> (-70, 34.05)
  line L9 (-70, 34.05) -> (-70.356, 34.0189)
  line L10 (-70.356, 34.0189) -> (-70.7011, 33.9264)
  line L11 (-70.7011, 33.9264) -> (-71.025, 33.7754)
  line L12 (-71.025, 33.7754) -> (-71.3177, 33.5704)
  line L13 (-71.3177, 33.5704) -> (-71.5704, 33.3177)
  line L14 (-71.5704, 33.3177) -> (-71.7754, 33.025)
  line L15 (-71.7754, 33.025) -> (-71.9264, 32.7011)
  line L16 (-71.9264, 32.7011) -> (-72.0189, 32.356)
  line L17 (-72.0189, 32.356) -> (-72.05, 32)
  line L18 (-72.05, 32) -> (-72.0189, 31.644)
  line L19 (-72.0189, 31.644) -> (-71.9264, 31.2989)
  line L20 (-71.9264, 31.2989) -> (-71.7754, 30.975)
  line L21 (-71.7754, 30.975) -> (-71.5704, 30.6823)
  line L22 (-71.5704, 30.6823) -> (-71.3177, 30.4296)
  line L23 (-71.3177, 30.4296) -> (-71.025, 30.2246)
  line L24 (-71.025, 30.2246) -> (-70.7011, 30.0736)
  line L25 (-70.7011, 30.0736) -> (-70.356, 29.9811)
  line L26 (-70.356, 29.9811) -> (-70, 29.95)
  line L27 (-70, 29.95) -> (-69.644, 29.9811)
  line L28 (-69.644, 29.9811) -> (-69.2989, 30.0736)
  line L29 (-69.2989, 30.0736) -> (-68.975, 30.2246)
  line L30 (-68.975, 30.2246) -> (-68.6823, 30.4296)
  line L31 (-68.6823, 30.4296) -> (-68.45, 30.6823)
  line L32 (-68.45, 30.6823) -> (-68.45, 30.975)
  line L33 (-68.45, 30.975) -> (-68.45, 31.2989)
  line L34 (-68.45, 31.2989) -> (-68.45, 31.644)
  line L35 (-68.45, 31.644) -> (-68.45, 32)
  circle A1 centre (-57, 32) radius 4
  circle A2 centre (-65.9828, 44.3637) radius 4
  circle A3 centre (-80.5172, 39.6412) radius 4
  circle A4 centre (-80.5172, 24.3588) radius 4
  circle A5 centre (-65.9828, 19.6363) radius 4
extrude "Extrude1'''''''''''''''''''''''''''''''''''''''''''''''''''''''''''" add sketch "Wheel_Hub_PETG_Rear_R" along normal blind 16 from surface at 62 separate body makes body 60 in component "Wheel_Hub_PETG_Rear_R"
sketch "Wheel_Tyre_TPU_Rear_R" plane through (0, 0, 0) normal (1, 0, 0) x (0, 0, -1) in component "Wheel_Tyre_TPU_Rear_R"
  circle A0 centre (-70, 32) radius 32
  circle A1 centre (-70, 32) radius 22
extrude "Extrude1''''''''''''''''''''''''''''''''''''''''''''''''''''''''''''" add sketch "Wheel_Tyre_TPU_Rear_R" along normal blind 16 from surface at 62 separate body makes body 61 in component "Wheel_Tyre_TPU_Rear_R"
sketch "Sketch1 (22)" plane through (0, 0, 0) normal (0, 1, 0) x (1, 0, 0) in component "3S_850mAh_LiPo_ENVELOPE_75x35x25"
  line L0 (-37.5, -38) -> (37.5, -38)
  line L1 (37.5, -38) -> (37.5, -3)
  line L2 (37.5, -3) -> (-37.5, -3)
  line L3 (-37.5, -3) -> (-37.5, -38)
extrude "Extrude1'''''''''''''''''''''''''''''''''''''''''''''''''''''''''''''" add sketch "Sketch1 (22)" along normal blind 25 from surface at 8 separate body makes body 62 in component "3S_850mAh_LiPo_ENVELOPE_75x35x25"
sketch "Sketch1 (23)" plane through (0, 0, 0) normal (0, 1, 0) x (1, 0, 0) in component "Skywalker_40A_ESC_55x25x12"
  line L0 (-60, -40) -> (-5, -40)
  line L1 (-5, -40) -> (-5, -15)
  line L2 (-5, -15) -> (-60, -15)
  line L3 (-60, -15) -> (-60, -40)
extrude "Extrude1''''''''''''''''''''''''''''''''''''''''''''''''''''''''''''''" add sketch "Sketch1 (23)" along normal blind 12 from surface at 34 separate body makes body 63 in component "Skywalker_40A_ESC_55x25x12"
sketch "Sketch1 (24)" plane through (0, 0, 0) normal (0, 1, 0) x (1, 0, 0) in component "ESP32_DevKit_51.5x28.3"
  line L0 (4, -42) -> (55.5, -42)
  line L1 (55.5, -42) -> (55.5, -13.7)
  line L2 (55.5, -13.7) -> (4, -13.7)
  line L3 (4, -13.7) -> (4, -42)
extrude "Extrude1'''''''''''''''''''''''''''''''''''''''''''''''''''''''''''''''" add sketch "Sketch1 (24)" along normal blind 14 from surface at 34 separate body makes body 64 in component "ESP32_DevKit_51.5x28.3"
sketch "Sketch1 (25)" plane through (0, 0, 0) normal (0, 1, 0) x (1, 0, 0) in component "DRV8871_L"
  line L0 (39, -45) -> (59, -45)
  line L1 (59, -45) -> (59, -25)
  line L2 (59, -25) -> (39, -25)
  line L3 (39, -25) -> (39, -45)
extrude "Extrude1''''''''''''''''''''''''''''''''''''''''''''''''''''''''''''''''" add sketch "Sketch1 (25)" along normal blind 6 from surface at 8 separate body makes body 65 in component "DRV8871_L"
sketch "Sketch1 (26)" plane through (0, 0, 0) normal (0, 1, 0) x (1, 0, 0) in component "DRV8871_R"
  line L0 (39, -24) -> (59, -24)
  line L1 (59, -24) -> (59, -4)
  line L2 (59, -4) -> (39, -4)
  line L3 (39, -4) -> (39, -24)
extrude "Extrude1'''''''''''''''''''''''''''''''''''''''''''''''''''''''''''''''''" add sketch "Sketch1 (26)" along normal blind 6 from surface at 8 separate body makes body 66 in component "DRV8871_R"
sketch "Sketch1 (27)" plane through (0, 0, 0) normal (0, 1, 0) x (1, 0, 0) in component "IMU_Foam_Pad_1mm"
  line L0 (-10.5, -56) -> (10.5, -56)
  line L1 (10.5, -56) -> (10.5, -40)
  line L2 (10.5, -40) -> (-10.5, -40)
  line L3 (-10.5, -40) -> (-10.5, -56)
extrude "Extrude1''''''''''''''''''''''''''''''''''''''''''''''''''''''''''''''''''" add sketch "Sketch1 (27)" along normal blind 1 from surface at 7 separate body makes body 67 in component "IMU_Foam_Pad_1mm"
sketch "Sketch1 (28)" plane through (0, 0, 0) normal (0, 1, 0) x (1, 0, 0) in component "IMU_GY521_MPU6050_21x16"
  line L0 (-10.5, -56) -> (10.5, -56)
  line L1 (10.5, -56) -> (10.5, -40)
  line L2 (10.5, -40) -> (-10.5, -40)
  line L3 (-10.5, -40) -> (-10.5, -56)
extrude "Extrude1'''''''''''''''''''''''''''''''''''''''''''''''''''''''''''''''''''" add sketch "Sketch1 (28)" along normal blind 3.5 from surface at 8 separate body makes body 68 in component "IMU_GY521_MPU6050_21x16"
sketch "Sketch1 (29)" plane through (0, 0, 0) normal (0, 1, 0) x (1, 0, 0) in component "Hall_Post_PETG"
  line L0 (8, 40) -> (12, 40)
  line L1 (12, 40) -> (12, 48)
  line L2 (12, 48) -> (8, 48)
  line L3 (8, 48) -> (8, 40)
extrude "Extrude1''''''''''''''''''''''''''''''''''''''''''''''''''''''''''''''''''''" add sketch "Sketch1 (29)" along normal blind 36 from surface at 7 separate body makes body 69 in component "Hall_Post_PETG"
sketch "Sketch1 (30)" plane through (0, 0, 0) normal (0, 1, 0) x (1, 0, 0) in component "Hall_A3144_TO92"
  line L0 (6.5, 42) -> (8, 42)
  line L1 (8, 42) -> (8, 46)
  line L2 (8, 46) -> (6.5, 46)
  line L3 (6.5, 46) -> (6.5, 42)
extrude "Extrude1'''''''''''''''''''''''''''''''''''''''''''''''''''''''''''''''''''''" add sketch "Sketch1 (30)" along normal blind 4 from surface at 37 separate body makes body 70 in component "Hall_A3144_TO92"
sketch "Sketch1 (31)" plane through (0, 0, 0) normal (0, 1, 0) x (1, 0, 0) in component "Power_Switch_Link"
  line L0 (66, -34) -> (80, -34)
  line L1 (80, -34) -> (80, -26)
  line L2 (80, -26) -> (66, -26)
  line L3 (66, -26) -> (66, -34)
extrude "Extrude1''''''''''''''''''''''''''''''''''''''''''''''''''''''''''''''''''''''" add sketch "Sketch1 (31)" along normal blind 10 from surface at 20 separate body makes body 71 in component "Power_Switch_Link"
component "01_Printed_Chassis_TPU" placed x (1, 0, 0) y (0, 1, 0) z (0, 0, 1) at (0, 0, 0)
component "02_Weapon_Beater" placed x (1, 0, 0) y (0, 1, 0) z (0, 0, 1) at (0, 0, 0)
component "03_Hinged_Wedgelets" placed x (1, 0, 0) y (0, 1, 0) z (0, 0, 1) at (0, 0, 0)
component "03b_Hinged_Skirts" placed x (1, 0, 0) y (0, 1, 0) z (0, 0, 1) at (0, 0, 0)
component "04_Drive_4WD" placed x (1, 0, 0) y (0, 1, 0) z (0, 0, 1) at (0, 0, 0)
component "05_Electronics_ENVELOPES" placed x (1, 0, 0) y (0, 1, 0) z (0, 0, 1) at (0, 0, 0)
component "Tub_TPU" placed x (1, 0, 0) y (0, 1, 0) z (0, 0, 1) at (0, 0, 0) in component "01_Printed_Chassis_TPU"
component "Lid_TPU_2mm" placed x (1, 0, 0) y (0, 1, 0) z (0, 0, 1) at (0, 0, 0) in component "01_Printed_Chassis_TPU"
component "Upright_6061_6mm_L" placed x (1, 0, 0) y (0, 1, 0) z (0, 0, 1) at (0, 0, 0) in component "02_Weapon_Beater"
component "Upright_6061_6mm_R" placed x (1, 0, 0) y (0, 1, 0) z (0, 0, 1) at (0, 0, 0) in component "02_Weapon_Beater"
component "Weapon_Top_Brace_3mm" placed x (1, 0, 0) y (0, 1, 0) z (0, 0, 1) at (0, 0, 0) in component "02_Weapon_Beater"
component "Weapon_Bottom_Brace_3mm" placed x (1, 0, 0) y (0, 1, 0) z (0, 0, 1) at (0, 0, 0) in component "02_Weapon_Beater"
component "Beater_Disc_L" placed x (1, 0, 0) y (0, 1, 0) z (0, 0, 1) at (0, 0, 0) in component "02_Weapon_Beater"
component "Beater_Disc_R" placed x (1, 0, 0) y (0, 1, 0) z (0, 0, 1) at (0, 0, 0) in component "02_Weapon_Beater"
component "Beater_Hub_6061_D30" placed x (1, 0, 0) y (0, 1, 0) z (0, 0, 1) at (0, 0, 0) in component "02_Weapon_Beater"
component "Bearing_608_L" placed x (1, 0, 0) y (0, 1, 0) z (0, 0, 1) at (0, 0, 0) in component "02_Weapon_Beater"
component "Bearing_608_R" placed x (1, 0, 0) y (0, 1, 0) z (0, 0, 1) at (0, 0, 0) in component "02_Weapon_Beater"
component "Spacer_Outer_L_ID8.2_OD11" placed x (1, 0, 0) y (0, 1, 0) z (0, 0, 1) at (0, 0, 0) in component "02_Weapon_Beater"
component "Spacer_Inner_ID8.2_OD11" placed x (1, 0, 0) y (0, 1, 0) z (0, 0, 1) at (0, 0, 0) in component "02_Weapon_Beater"
component "Spacer_Outer_R_ID8.2_OD11" placed x (1, 0, 0) y (0, 1, 0) z (0, 0, 1) at (0, 0, 0) in component "02_Weapon_Beater"
component "Dead_Shaft_M8_12.9" placed x (1, 0, 0) y (0, 1, 0) z (0, 0, 1) at (0, 0, 0) in component "02_Weapon_Beater"
component "D3536_1250kV_Can_ENVELOPE" placed x (1, 0, 0) y (0, 1, 0) z (0, 0, 1) at (0, 0, 0) in component "02_Weapon_Beater"
component "Motor_Pulley_D26_Groove" placed x (1, 0, 0) y (0, 1, 0) z (0, 0, 1) at (0, 0, 0) in component "02_Weapon_Beater"
component "Weapon_Motor_Mount_3mm" placed x (1, 0, 0) y (0, 1, 0) z (0, 0, 1) at (0, 0, 0) in component "02_Weapon_Beater"
component "Belt_Upper_ENVELOPE" placed x (1, 0, 0) y (0, 1, 0) z (0, 0, 1) at (0, 0, 0) in component "02_Weapon_Beater"
component "Belt_Lower_ENVELOPE" placed x (1, 0, 0) y (0, 1, 0) z (0, 0, 1) at (0, 0, 0) in component "02_Weapon_Beater"
component "Wedgelet_L" placed x (1, 0, 0) y (0, 1, 0) z (0, 0, 1) at (0, 0, 0) in component "03_Hinged_Wedgelets"
component "Wedgelet_R" placed x (1, 0, 0) y (0, 1, 0) z (0, 0, 1) at (0, 0, 0) in component "03_Hinged_Wedgelets"
component "Wedgelet_Block_PETG_L" placed x (1, 0, 0) y (0, 1, 0) z (0, 0, 1) at (0, 0, 0) in component "03_Hinged_Wedgelets"
component "Wedgelet_Carrier_PETG_L1" placed x (1, 0, 0) y (0, 1, 0) z (0, 0, 1) at (0, 0, 0) in component "03_Hinged_Wedgelets"
component "Wedgelet_Carrier_PETG_L2" placed x (1, 0, 0) y (0, 1, 0) z (0, 0, 1) at (0, 0, 0) in component "03_Hinged_Wedgelets"
component "Hinge_Pin_D3_L" placed x (1, 0, 0) y (0, 1, 0) z (0, 0, 1) at (0, 0, 0) in component "03_Hinged_Wedgelets"
component "Eclip_DIN6799_2.3_L" placed x (1, 0, 0) y (0, 1, 0) z (0, 0, 1) at (0, 0, 0) in component "03_Hinged_Wedgelets"
component "Wedgelet_Block_PETG_R" placed x (1, 0, 0) y (0, 1, 0) z (0, 0, 1) at (0, 0, 0) in component "03_Hinged_Wedgelets"
component "Wedgelet_Carrier_PETG_R1" placed x (1, 0, 0) y (0, 1, 0) z (0, 0, 1) at (0, 0, 0) in component "03_Hinged_Wedgelets"
component "Wedgelet_Carrier_PETG_R2" placed x (1, 0, 0) y (0, 1, 0) z (0, 0, 1) at (0, 0, 0) in component "03_Hinged_Wedgelets"